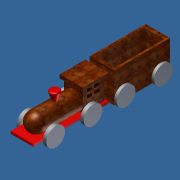
# Autodesk Inventor part: trainRed
Saved by Autodesk Inventor 2012 (Build 160160000, 160)
## iProperties
Created: 2015-09-05
Part Number: trainRed
Material: Default
Document SubType Name: Modeling
Designer: Chris
Density: 1 g/cm^3
Author: Chris
Autodesk Inventor part; units mm, degrees
sketch "Sketch1" plane through (0, 0, 0) normal (0, 0, 1) x (1, 0, 0)
  circle A0 centre (0, 0) radius 50.8
  dimension "d6" = 101.6
  constraints: 1 centre point
  measures "d6" diameter of A0
extrude "Extrusion1" add sketch "Sketch1" along normal blind 254
fillet "Fillet1" radius 50.8 1 edges at (-50.8, 0, 254)
ref_plane "Work Plane1" through (0, 0, 101.6) normal (0, 0, -1) x (-1, 0, 0)
sketch "Sketch2" plane through (0, 0, 101.6) normal (0, 0, -1) x (-1, 0, 0)
  line L0 (-11.7457, 49.4574) -> (-28.5577, 98.2869)
  line L1 (-28.5577, 98.2869) -> (0, 98.2869)
  arc A0 (0, 50.8477) -> (-11.7457, 49.4574) centre (-0.1993, 2.2226) ccw
  line L2 (0, 50.8477) -> (0, 98.2869)
  point P0 (0, 0)
  constraints: 6 end point, 2 point on circle, 1 centre point, 1 horizontal, 1 perpendicular
revolve "Revolution1" add sketch "Sketch2" angle 360 about axis through (0, 50.8477, 101.6) along (0, 1, 0)
fillet "Fillet2" radius 6.35 1 edges at (-28.5577, 98.2869, 101.6)
sketch "Sketch6" plane through (0, 0, 0) normal (1, 0, 0) x (0, 1, 0)
  point P0 (0, 0)
ref_plane "Work Plane2" through (0, -38.1, 0) normal (0, 1, 0) x (-1, 0, 0)
sketch "Sketch7" plane through (0, -38.1, 0) normal (0, 1, 0) x (-1, 0, 0)
  line L0 (-61.9791, 279.4) -> (61.7849, 279.4)
  line L1 (61.7849, 279.4) -> (61.7849, -127)
  line L2 (61.7849, -127) -> (-61.9791, -127)
  line L3 (-61.9791, -127) -> (-61.9791, 279.4)
  line L4 (-50.8, 0) -> (50.8, 0) projected
  point P0 (0, 0)
  dimension "d28" = 279.4
  dimension "d29" = 127
  constraints: 8 end point, 2 parallel, 1 horizontal, 1 perpendicular
  measures "d28" distance between parallel lines of L0 L4
  measures "d29" distance between parallel lines of L2 L4
extrude "Extrusion3" add sketch "Sketch7" against normal blind 12.7
sketch "Sketch8" plane through (0, -38.1, 0) normal (0, 1, 0) x (1, 0, 0)
  line L0 (-51.0558, 114.9502) -> (51.9231, 114.9502)
  line L1 (51.9231, 114.9502) -> (51.9231, 0)
  line L2 (51.9231, 0) -> (-51.0558, 0)
  line L3 (-51.0558, 0) -> (-51.0558, 114.9502)
  point P0 (0, 0)
  constraints: 8 end point, 2 parallel, 1 horizontal, 1 perpendicular
extrude "Extrusion4" add sketch "Sketch8" along normal blind 114.3
sketch "Sketch9" plane through (0, 76.2, 0) normal (0, 1, 0) x (1, 0, 0)
  line L0 (-62.1613, 126.8007) -> (62.3556, 126.8007)
  line L1 (62.3556, 126.8007) -> (62.3556, -12.5236)
  line L2 (62.3556, -12.5236) -> (-62.1613, -12.5236)
  line L3 (-62.1613, -12.5236) -> (-62.1613, 126.8007)
  point P0 (0, 0)
  constraints: 8 end point, 2 parallel, 1 horizontal, 1 perpendicular
extrude "Extrusion5" add sketch "Sketch9" along normal blind 19.05
sketch "Sketch10" plane through (61.9791, -38.1, 279.4) normal (1, 0, 0) x (0, 0, -1)
  line L0 (406.4, 0) -> (406.4, -12.7) projected
  line L1 (0, 0) -> (0, -12.7) projected
  circle A0 centre (101.6, -6.35) radius 50.8
  circle A1 centre (304.8, -6.35) radius 50.8
  point P0 (279.4, 38.1)
  dimension "d36" = 101.6
  dimension "d37" = 101.6
  dimension "d38" = 101.6
  dimension "d39" = 101.6
  constraints: 2 centre point
  measures "d36" diameter of A0
  measures "d37" diameter of A1
  measures "d38" distance from line of L1 A0.centre
  measures "d39" distance from line of L0 A1.centre
extrude "Extrusion6" add sketch "Sketch10" along normal blind 19.05
mirror "Mirror1" about plane through (0, 0, 0) normal (1, 0, 0) of "Extrusion6"
sketch "Sketch11" plane through (51.9231, -38.1, 0) normal (1, 0, 0) x (0, 0, -1)
  line L0 (21.6586, 105.4336) -> (48.3212, 105.4336)
  line L1 (48.3212, 105.4336) -> (48.3212, 82.0137)
  line L2 (48.3212, 82.0137) -> (21.6586, 82.0137)
  line L3 (21.6586, 82.0137) -> (21.6586, 105.4336)
  line L4 (61.6525, 105.4336) -> (89.396, 105.4336)
  line L5 (89.396, 105.4336) -> (89.396, 82.0137)
  line L6 (89.396, 82.0137) -> (61.6525, 82.0137)
  line L7 (61.6525, 82.0137) -> (61.6525, 105.4336)
  line L8 (21.6586, 73.7267) -> (48.3212, 73.7267)
  line L9 (48.3212, 73.7267) -> (48.3212, 52.829)
  line L10 (48.3212, 52.829) -> (21.6586, 52.829)
  line L11 (21.6586, 52.829) -> (21.6586, 73.7267)
  line L12 (61.6525, 73.7267) -> (89.396, 73.7267)
  line L13 (89.396, 73.7267) -> (89.396, 52.829)
  line L14 (89.396, 52.829) -> (61.6525, 52.829)
  line L15 (61.6525, 52.829) -> (61.6525, 73.7267)
  point P0 (0, 38.1)
  constraints: 32 end point, 8 parallel, 4 horizontal, 4 perpendicular
extrude "Extrusion7" cut sketch "Sketch11" against normal blind 6.35
mirror "Mirror2" about plane through (0, 0, 0) normal (1, 0, 0) of "Extrusion7"
ref_plane "Work Plane3" through (51.9231, -38.1, -153.0502) normal (0, 0, -1) x (-1, 0, 0)
sketch "Sketch12" plane through (51.9231, -38.1, -153.0502) normal (0, 0, -1) x (-1, 0, 0)
  line L0 (-15.2402, 133.3315) -> (118.0839, 133.3315)
  line L1 (118.0839, 133.3315) -> (118.0839, -31.0681)
  line L2 (118.0839, -31.0681) -> (-15.2402, -31.0681)
  line L3 (-15.2402, -31.0681) -> (-15.2402, 133.3315)
  point P0 (51.9231, 38.1)
  constraints: 8 end point, 2 parallel, 1 horizontal, 1 perpendicular
extrude "Extrusion8" add sketch "Sketch12" along normal blind 304.8
mirror "Mirror3" about plane through (-51.0558, -38.1, -114.9502) normal (0, 0, -1) of "Extrusion6"
mirror "Mirror4" about plane through (0, 0, 0) normal (1, 0, 0) of "Extrusion6", "Mirror3"
sketch "Sketch13" plane through (-66.1608, 95.2315, -153.0502) normal (0, 1, 0) x (1, 0, 0)
  line L0 (13.5794, 283.5214) -> (121.3059, 283.5214)
  line L1 (121.3059, 283.5214) -> (121.3059, 18.1085)
  line L2 (121.3059, 18.1085) -> (13.5794, 18.1085)
  line L3 (13.5794, 18.1085) -> (13.5794, 283.5214)
  point P0 (66.1608, -153.0502)
  constraints: 8 end point, 2 parallel, 1 horizontal, 1 perpendicular
extrude "Extrusion9" cut sketch "Sketch13" against normal blind 152.4
sketch "Sketch14" plane through (51.9231, -38.1, -153.0502) normal (0, 0, 1) x (1, 0, 0)
  line L0 (-69.6171, 4.1819) -> (-35.0132, 4.1819)
  line L1 (-35.0132, 4.1819) -> (-35.0132, -8.2696)
  line L2 (-35.0132, -8.2696) -> (-69.6171, -8.2696)
  line L3 (-69.6171, -8.2696) -> (-69.6171, 4.1819)
  point P0 (-51.9231, 38.1)
  constraints: 8 end point, 2 parallel, 1 horizontal, 1 perpendicular
extrude "Extrusion10" add sketch "Sketch14" along normal blind 50.8
body "Solid1"
